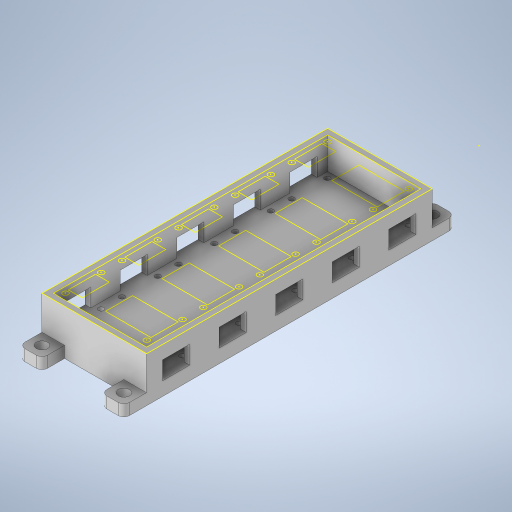
# Autodesk Inventor part: RelayCaseBottom
Saved by Autodesk Inventor 2024 (Build 280153000, 153)
## iProperties
Created: 2023-08-11
Part Number: RelayCaseBottom
Material: Generic
Document SubType Name: Modeling
Designer: 18179
Density: 1 g/cm^3
Appearance: Default
Autodesk Inventor part; units mm, degrees
ref_plane "YZ Plane" through (0, 0, 0) normal (1, 0, 0) x (0, 1, 0)
ref_plane "XZ Plane" through (0, 0, 0) normal (0, 1, 0) x (-1, 0, 0)
ref_plane "XY Plane" through (0, 0, 0) normal (0, 0, 1) x (1, 0, 0)
sketch "0" plane through (0, 0, 0) normal (0, 0, 1) x (1, 0, 0)
  line L0 (-39.8611, 34.3581) -> (-39.8611, 26.7381)
  line L1 (-39.8611, 26.7381) -> (-42.4011, 26.7381)
  line L2 (-42.4011, 26.7381) -> (-42.4011, 34.3581)
  line L3 (-42.4011, 34.3581) -> (-39.8611, 34.3581)
  line L4 (-37.9769, 46.974) -> (-63.3769, 46.974)
  line L5 (-63.3769, 46.974) -> (-63.3769, -3.826)
  line L6 (-63.3769, -3.826) -> (-37.9769, -3.826)
  line L7 (-37.9769, -3.826) -> (-37.9769, 46.974)
  line L8 (-58.2715, 6.588) -> (-58.2715, 24.368)
  line L9 (-58.2715, 24.368) -> (-43.0823, 24.368)
  line L10 (-43.0823, 24.368) -> (-43.0823, 6.588)
  line L11 (-43.0823, 6.588) -> (-43.0569, 6.588)
  line L12 (-43.0569, 6.588) -> (-43.0569, -1.159)
  line L13 (-43.0569, -1.159) -> (-58.2969, -1.159)
  line L14 (-58.2969, -1.159) -> (-58.2969, 6.588)
  line L15 (-58.2969, 6.588) -> (-58.2715, 6.588)
  line L16 (-58.2969, 37.449) -> (-58.2969, 45.196)
  line L17 (-58.2969, 45.196) -> (-43.0569, 45.196)
  line L18 (-43.0569, 45.196) -> (-43.0569, 37.449)
  line L19 (-43.0569, 37.449) -> (-58.2969, 37.449)
  circle A0 centre (-60.7099, -1.2407) radius 1.524
  circle A1 centre (-40.6439, -1.2407) radius 1.524
  circle A2 centre (-60.7099, 44.3888) radius 1.524
  circle A3 centre (-40.6439, 44.3888) radius 1.524
  line L20 (-71.6111, 34.3581) -> (-71.6111, 26.7381)
  line L21 (-71.6111, 26.7381) -> (-74.1511, 26.7381)
  line L22 (-74.1511, 26.7381) -> (-74.1511, 34.3581)
  line L23 (-74.1511, 34.3581) -> (-71.6111, 34.3581)
  line L24 (-69.7269, 46.974) -> (-95.1269, 46.974)
  line L25 (-95.1269, 46.974) -> (-95.1269, -3.826)
  line L26 (-95.1269, -3.826) -> (-69.7269, -3.826)
  line L27 (-69.7269, -3.826) -> (-69.7269, 46.974)
  line L28 (-90.0215, 6.588) -> (-90.0215, 24.368)
  line L29 (-90.0215, 24.368) -> (-74.8323, 24.368)
  line L30 (-74.8323, 24.368) -> (-74.8323, 6.588)
  line L31 (-74.8323, 6.588) -> (-74.8069, 6.588)
  line L32 (-74.8069, 6.588) -> (-74.8069, -1.159)
  line L33 (-74.8069, -1.159) -> (-90.0469, -1.159)
  line L34 (-90.0469, -1.159) -> (-90.0469, 6.588)
  line L35 (-90.0469, 6.588) -> (-90.0215, 6.588)
  line L36 (-90.0469, 37.449) -> (-90.0469, 45.196)
  line L37 (-90.0469, 45.196) -> (-74.8069, 45.196)
  line L38 (-74.8069, 45.196) -> (-74.8069, 37.449)
  line L39 (-74.8069, 37.449) -> (-90.0469, 37.449)
  circle A4 centre (-92.4599, -1.2407) radius 1.524
  circle A5 centre (-72.3939, -1.2407) radius 1.524
  circle A6 centre (-92.4599, 44.3888) radius 1.524
  circle A7 centre (-72.3939, 44.3888) radius 1.524
  line L40 (-103.3611, 34.3581) -> (-103.3611, 26.7381)
  line L41 (-103.3611, 26.7381) -> (-105.9011, 26.7381)
  line L42 (-105.9011, 26.7381) -> (-105.9011, 34.3581)
  line L43 (-105.9011, 34.3581) -> (-103.3611, 34.3581)
  line L44 (-101.4769, 46.974) -> (-126.8769, 46.974)
  line L45 (-126.8769, 46.974) -> (-126.8769, -3.826)
  line L46 (-126.8769, -3.826) -> (-101.4769, -3.826)
  line L47 (-101.4769, -3.826) -> (-101.4769, 46.974)
  line L48 (-121.7715, 6.588) -> (-121.7715, 24.368)
  line L49 (-121.7715, 24.368) -> (-106.5823, 24.368)
  line L50 (-106.5823, 24.368) -> (-106.5823, 6.588)
  line L51 (-106.5823, 6.588) -> (-106.5569, 6.588)
  line L52 (-106.5569, 6.588) -> (-106.5569, -1.159)
  line L53 (-106.5569, -1.159) -> (-121.7969, -1.159)
  line L54 (-121.7969, -1.159) -> (-121.7969, 6.588)
  line L55 (-121.7969, 6.588) -> (-121.7715, 6.588)
  line L56 (-121.7969, 37.449) -> (-121.7969, 45.196)
  line L57 (-121.7969, 45.196) -> (-106.5569, 45.196)
  line L58 (-106.5569, 45.196) -> (-106.5569, 37.449)
  line L59 (-106.5569, 37.449) -> (-121.7969, 37.449)
  circle A8 centre (-124.2099, -1.2407) radius 1.524
  circle A9 centre (-104.1439, -1.2407) radius 1.524
  circle A10 centre (-124.2099, 44.3888) radius 1.524
  circle A11 centre (-104.1439, 44.3888) radius 1.524
  line L60 (-135.1111, 34.3581) -> (-135.1111, 26.7381)
  line L61 (-135.1111, 26.7381) -> (-137.6511, 26.7381)
  line L62 (-137.6511, 26.7381) -> (-137.6511, 34.3581)
  line L63 (-137.6511, 34.3581) -> (-135.1111, 34.3581)
  line L64 (-133.2269, 46.974) -> (-158.6269, 46.974)
  line L65 (-158.6269, 46.974) -> (-158.6269, -3.826)
  line L66 (-158.6269, -3.826) -> (-133.2269, -3.826)
  line L67 (-133.2269, -3.826) -> (-133.2269, 46.974)
  line L68 (-153.5215, 6.588) -> (-153.5215, 24.368)
  line L69 (-153.5215, 24.368) -> (-138.3323, 24.368)
  line L70 (-138.3323, 24.368) -> (-138.3323, 6.588)
  line L71 (-138.3323, 6.588) -> (-138.3069, 6.588)
  line L72 (-138.3069, 6.588) -> (-138.3069, -1.159)
  line L73 (-138.3069, -1.159) -> (-153.5469, -1.159)
  line L74 (-153.5469, -1.159) -> (-153.5469, 6.588)
  line L75 (-153.5469, 6.588) -> (-153.5215, 6.588)
  line L76 (-153.5469, 37.449) -> (-153.5469, 45.196)
  line L77 (-153.5469, 45.196) -> (-138.3069, 45.196)
  line L78 (-138.3069, 45.196) -> (-138.3069, 37.449)
  line L79 (-138.3069, 37.449) -> (-153.5469, 37.449)
  circle A12 centre (-155.9599, -1.2407) radius 1.524
  circle A13 centre (-135.8939, -1.2407) radius 1.524
  circle A14 centre (-155.9599, 44.3888) radius 1.524
  circle A15 centre (-135.8939, 44.3888) radius 1.524
  line L80 (-166.8611, 34.3581) -> (-166.8611, 26.7381)
  line L81 (-166.8611, 26.7381) -> (-169.4011, 26.7381)
  line L82 (-169.4011, 26.7381) -> (-169.4011, 34.3581)
  line L83 (-169.4011, 34.3581) -> (-166.8611, 34.3581)
  line L84 (-164.9769, 46.974) -> (-190.3769, 46.974)
  line L85 (-190.3769, 46.974) -> (-190.3769, -3.826)
  line L86 (-190.3769, -3.826) -> (-164.9769, -3.826)
  line L87 (-164.9769, -3.826) -> (-164.9769, 46.974)
  line L88 (-185.2715, 6.588) -> (-185.2715, 24.368)
  line L89 (-185.2715, 24.368) -> (-170.0823, 24.368)
  line L90 (-170.0823, 24.368) -> (-170.0823, 6.588)
  line L91 (-170.0823, 6.588) -> (-170.0569, 6.588)
  line L92 (-170.0569, 6.588) -> (-170.0569, -1.159)
  line L93 (-170.0569, -1.159) -> (-185.2969, -1.159)
  line L94 (-185.2969, -1.159) -> (-185.2969, 6.588)
  line L95 (-185.2969, 6.588) -> (-185.2715, 6.588)
  line L96 (-185.2969, 37.449) -> (-185.2969, 45.196)
  line L97 (-185.2969, 45.196) -> (-170.0569, 45.196)
  line L98 (-170.0569, 45.196) -> (-170.0569, 37.449)
  line L99 (-170.0569, 37.449) -> (-185.2969, 37.449)
  circle A16 centre (-187.7099, -1.2407) radius 1.524
  circle A17 centre (-167.6439, -1.2407) radius 1.524
  circle A18 centre (-187.7099, 44.3888) radius 1.524
  circle A19 centre (-167.6439, 44.3888) radius 1.524
  line L100 (-37.9769, -3.826) -> (-190.3769, -3.826)
  line L101 (-190.3769, -3.826) -> (-190.3769, 46.974)
  line L102 (-190.3769, 46.974) -> (-37.9769, 46.974)
  line L103 (-37.9769, 46.974) -> (-37.9769, -3.826)
  line L104 (-190.3769, 47.736) -> (-37.2149, 47.736)
  line L105 (-37.2149, 47.736) -> (-37.2149, -3.826)
  line L106 (-37.9769, -4.588) -> (-191.1389, -4.588)
  line L107 (-191.1389, -4.588) -> (-191.1389, 46.974)
  line L108 (-191.1389, -4.588) -> (-37.2149, -4.588)
  line L109 (-37.2149, -4.588) -> (-37.2149, 47.736)
  line L110 (-37.2149, 47.736) -> (-191.1389, 47.736)
  line L111 (-191.1389, 47.736) -> (-191.1389, -4.588)
  point P0 (-37.2149, -3.826)
  dimension "d0" = 25.4
  dimension "d1" = 50.8
  dimension "d2" = 3.048
  dimension "d3" = 1.8843
  dimension "d4" = 4.4243
  dimension "d5" = 5.08
  dimension "d6" = 5.08
  dimension "d7" = 5.1054
  dimension "d8" = 20.2946
  dimension "d9" = 20.32
  dimension "d10" = 20.32
  dimension "d11" = 7.62
  dimension "d12" = 12.6159
  dimension "d13" = 10.8379
  dimension "d14" = 3.0909
  dimension "d15" = 9.9901
  dimension "d16" = 35.5171
  dimension "d17" = 27.7701
  dimension "d18" = 20.1501
  dimension "d19" = 12.6159
  dimension "d20" = 0
  dimension "d21" = 38.1841
  dimension "d22" = 0
  dimension "d23" = 0
  dimension "d24" = 1.8843
  dimension "d25" = 7.62
  dimension "d26" = 1.8843
  dimension "d27" = 2.667
  dimension "d28" = 10.0307
  dimension "d29" = 2.667
  dimension "d30" = 35.5988
  dimension "d31" = 0
  dimension "d32" = 4.4243
  dimension "d33" = 7.62
  dimension "d34" = 4.4243
  dimension "d35" = 10.8379
  dimension "d36" = 5.08
  dimension "d37" = 3.0909
  dimension "d38" = 5.08
  dimension "d39" = 5.08
  dimension "d40" = 27.7701
  dimension "d41" = 5.08
  dimension "d42" = 35.5171
  dimension "d43" = 9.9901
  dimension "d44" = 5.1054
  dimension "d45" = 5.1054
  dimension "d46" = 27.7701
  dimension "d47" = 9.9901
  dimension "d48" = 20.2946
  dimension "d49" = 27.7701
  dimension "d50" = 20.2946
  dimension "d51" = 10.8379
  dimension "d52" = 20.32
  dimension "d53" = 3.0909
  dimension "d54" = 20.32
  dimension "d55" = 20.32
  dimension "d56" = 27.7701
  dimension "d57" = 20.32
  dimension "d58" = 35.5171
  dimension "d59" = 22.733
  dimension "d60" = 10.0307
  dimension "d61" = 22.733
  dimension "d62" = 35.5988
  dimension "d63" = 25.4
  constraints: 224 end point, 44 parallel, 38 perpendicular, 20 centre point, 15 equal radius, 14 collinear, 2 horizontal, 2 other
  measures "d0" distance between parallel lines of L7 L5
  measures "d1" distance between parallel lines of L6 L4
  measures "d2" diameter of A3
  measures "d3" distance between parallel lines of L0 L7
  measures "d4" distance between parallel lines of L2 L7
  measures "d5" distance between parallel lines of L7 L18
  measures "d6" distance between parallel lines of L12 L7
  measures "d7" distance between parallel lines of L7 L10
  measures "d8" distance between parallel lines of L7 L8
  measures "d9" distance between parallel lines of L7 L16
  measures "d10" distance between parallel lines of L14 L7
  measures "d11" distance between parallel lines of L1 L3
  measures "d12" distance between parallel lines of L3 L4
  measures "d13" distance between parallel lines of L3 L17
  measures "d14" distance between parallel lines of L3 L19
  measures "d15" distance between parallel lines of L3 L9
  measures "d16" distance between parallel lines of L13 L3
  measures "d17" distance between parallel lines of L3 L15
  measures "d18" distance between parallel lines of L11 L1
  measures "d19" distance from line of L7.end L3
  measures "d20" distance from line of L4.start L7
  measures "d21" distance from line of L7.start L3
  measures "d22" distance from line of L6.end L7
  measures "d23" distance from line of L0.start L3
  measures "d24" distance from line of L3.end L7
  measures "d25" distance from line of L0.end L3
  measures "d26" distance from line of L1.start L7
  measures "d27" distance from line of A3.centre L7
  measures "d28" distance from line of A3.centre L3
  measures "d29" distance from line of A1.centre L7
  measures "d30" distance from line of A1.centre L3
  measures "d31" distance from line of L2.end L3
  measures "d32" distance from line of L3.start L7
  measures "d33" distance from line of L2.start L3
  measures "d34" distance from line of L1.end L7
  measures "d35" distance from line of L18.start L3
  measures "d36" distance from line of L17.end L7
  measures "d37" distance from line of L18.end L3
  measures "d38" distance from line of L19.start L7
  measures "d39" distance from line of L11.end L7
  measures "d40" distance from line of L12.start L3
  measures "d41" distance from line of L13.start L7
  measures "d42" distance from line of L12.end L3
  measures "d43" distance from line of L10.start L3
  measures "d44" distance from line of L9.end L7
  measures "d45" distance from line of L11.start L7
  measures "d46" distance from line of L10.end L3
  measures "d47" distance from line of L8.end L3
  measures "d48" distance from line of L9.start L7
  measures "d49" distance from line of L8.start L3
  measures "d50" distance from line of L15.end L7
  measures "d51" distance from line of L16.end L3
  measures "d52" distance from line of L17.start L7
  measures "d53" distance from line of L16.start L3
  measures "d54" distance from line of L19.end L7
  measures "d55" distance from line of L15.start L7
  measures "d56" distance from line of L14.end L3
  measures "d57" distance from line of L13.end L7
  measures "d58" distance from line of L14.start L3
  measures "d59" distance from line of A2.centre L7
  measures "d60" distance from line of A2.centre L3
  measures "d61" distance from line of A0.centre L7
  measures "d62" distance from line of A0.centre L3
  measures "d63" distance from line of L4.end L7
extrude "Extrusion1" add sketch "0" along normal blind 3.175 contours L0 L1 L2 L3 | L7 L6 L5 L4 | L5 L100 L27 L102 | L27 L26 L25 L24 | L25 L100 L47 L102 | L47 L46 L45 L44 | L45 L100 L67 L102 | L67 L66 L65 L64 | L65 L100 L87 L102 | L87 L86 L85 L84 | L20 L21 L22 L23 | L40 L41 L42 L43 | L60 L61 L62 L63 | L80 L81 L82 L83 | L104 L105 L109 L108 L106 L107 L111 L110
sketch "Sketch3" plane through (0, 0, 3.175) normal (0, 0, 1) x (1, 0, 0)
  line L0 (-191.1389, 47.736) -> (-191.1389, -4.588) projected
  line L1 (-191.1389, -4.588) -> (-37.2149, -4.588) projected
  line L2 (-37.2149, -4.588) -> (-37.2149, 47.736) projected
  line L3 (-37.2149, 47.736) -> (-191.1389, 47.736) projected
  line L4 (-58.2969, 37.449) -> (-58.2969, 45.196) projected
  line L5 (-58.2969, 45.196) -> (-43.0569, 45.196) projected
  line L6 (-43.0569, 45.196) -> (-43.0569, 37.449) projected
  line L7 (-43.0569, 37.449) -> (-58.2969, 37.449) projected
  circle A0 centre (-40.6439, 44.3888) radius 1.524 projected
  circle A1 centre (-60.7099, 44.3888) radius 1.524 projected
  circle A2 centre (-40.6439, -1.2407) radius 1.524 projected
  circle A3 centre (-60.7099, -1.2407) radius 1.524 projected
  line L8 (-106.5569, 37.449) -> (-121.7969, 37.449) projected
  line L9 (-121.7969, 37.449) -> (-121.7969, 45.196) projected
  line L10 (-121.7969, 45.196) -> (-106.5569, 45.196) projected
  line L11 (-106.5569, 45.196) -> (-106.5569, 37.449) projected
  circle A4 centre (-124.2099, 44.3888) radius 1.524 projected
  circle A5 centre (-104.1439, 44.3888) radius 1.524 projected
  circle A6 centre (-124.2099, -1.2407) radius 1.524 projected
  circle A7 centre (-104.1439, -1.2407) radius 1.524 projected
  circle A8 centre (-167.6439, -1.2407) radius 1.524 projected
  circle A9 centre (-187.7099, -1.2407) radius 1.524 projected
  circle A10 centre (-167.6439, 44.3888) radius 1.524 projected
  circle A11 centre (-187.7099, 44.3888) radius 1.524 projected
  line L12 (-170.0569, 37.449) -> (-185.2969, 37.449) projected
  line L13 (-185.2969, 37.449) -> (-185.2969, 45.196) projected
  line L14 (-185.2969, 45.196) -> (-170.0569, 45.196) projected
  line L15 (-170.0569, 45.196) -> (-170.0569, 37.449) projected
  line L16 (-185.2969, -1.159) -> (-185.2969, 6.588) projected
  line L17 (-185.2969, 6.588) -> (-185.2715, 6.588) projected
  line L18 (-185.2715, 6.588) -> (-185.2715, 24.368) projected
  line L19 (-185.2715, 24.368) -> (-170.0823, 24.368) projected
  line L20 (-170.0823, 24.368) -> (-170.0823, 6.588) projected
  line L21 (-170.0823, 6.588) -> (-170.0569, 6.588) projected
  line L22 (-170.0569, 6.588) -> (-170.0569, -1.159) projected
  line L23 (-170.0569, -1.159) -> (-185.2969, -1.159) projected
  circle A12 centre (-135.8939, -1.2407) radius 1.524 projected
  circle A13 centre (-155.9599, -1.2407) radius 1.524 projected
  circle A14 centre (-135.8939, 44.3888) radius 1.524 projected
  circle A15 centre (-155.9599, 44.3888) radius 1.524 projected
  line L24 (-138.3069, 37.449) -> (-153.5469, 37.449) projected
  line L25 (-153.5469, 37.449) -> (-153.5469, 45.196) projected
  line L26 (-153.5469, 45.196) -> (-138.3069, 45.196) projected
  line L27 (-138.3069, 45.196) -> (-138.3069, 37.449) projected
  circle A16 centre (-72.3939, -1.2407) radius 1.524 projected
  circle A17 centre (-92.4599, -1.2407) radius 1.524 projected
  circle A18 centre (-72.3939, 44.3888) radius 1.524 projected
  circle A19 centre (-92.4599, 44.3888) radius 1.524 projected
  line L28 (-74.8069, 37.449) -> (-90.0469, 37.449) projected
  line L29 (-90.0469, 37.449) -> (-90.0469, 45.196) projected
  line L30 (-90.0469, 45.196) -> (-74.8069, 45.196) projected
  line L31 (-74.8069, 45.196) -> (-74.8069, 37.449) projected
  line L32 (-194.3139, 50.911) -> (-194.3139, -7.763)
  line L33 (-194.3139, -7.763) -> (-34.0399, -7.763)
  line L34 (-34.0399, -7.763) -> (-34.0399, 50.911)
  line L35 (-34.0399, 50.911) -> (-194.3139, 50.911)
  line L36 (-185.2969, 45.196) -> (-170.0569, 45.196)
  line L37 (-170.0569, 45.196) -> (-170.0569, 50.911)
  line L38 (-170.0569, 50.911) -> (-185.2969, 50.911)
  line L39 (-185.2969, 50.911) -> (-185.2969, 45.196)
  line L40 (-153.5469, 45.196) -> (-138.3069, 45.196)
  line L41 (-138.3069, 45.196) -> (-138.3069, 50.911)
  line L42 (-138.3069, 50.911) -> (-153.5469, 50.911)
  line L43 (-153.5469, 50.911) -> (-153.5469, 45.196)
  line L44 (-121.7969, 45.196) -> (-106.5569, 45.196)
  line L45 (-106.5569, 45.196) -> (-106.5569, 50.911)
  line L46 (-106.5569, 50.911) -> (-121.7969, 50.911)
  line L47 (-121.7969, 50.911) -> (-121.7969, 45.196)
  line L48 (-90.0469, 45.196) -> (-74.8069, 45.196)
  line L49 (-74.8069, 45.196) -> (-74.8069, 50.911)
  line L50 (-74.8069, 50.911) -> (-90.0469, 50.911)
  line L51 (-90.0469, 50.911) -> (-90.0469, 45.196)
  line L52 (-58.2969, 45.196) -> (-43.0569, 45.196)
  line L53 (-43.0569, 45.196) -> (-43.0569, 50.911)
  line L54 (-43.0569, 50.911) -> (-58.2969, 50.911)
  line L55 (-58.2969, 50.911) -> (-58.2969, 45.196)
  line L56 (-185.2969, 50.911) -> (-170.0569, 50.911)
  line L57 (-170.0569, 50.911) -> (-170.0569, -7.763)
  line L58 (-170.0569, -7.763) -> (-185.2969, -7.763)
  line L59 (-185.2969, -7.763) -> (-185.2969, 50.911)
  line L60 (-153.5469, 50.911) -> (-138.3069, 50.911)
  line L61 (-138.3069, 50.911) -> (-138.3069, -7.763)
  line L62 (-138.3069, -7.763) -> (-153.5469, -7.763)
  line L63 (-153.5469, -7.763) -> (-153.5469, 50.911)
  line L64 (-121.7969, 50.911) -> (-106.5569, 50.911)
  line L65 (-106.5569, 50.911) -> (-106.5569, -7.763)
  line L66 (-106.5569, -7.763) -> (-121.7969, -7.763)
  line L67 (-121.7969, -7.763) -> (-121.7969, 50.911)
  line L68 (-90.0469, 50.911) -> (-74.8069, 50.911)
  line L69 (-74.8069, 50.911) -> (-74.8069, -7.763)
  line L70 (-74.8069, -7.763) -> (-90.0469, -7.763)
  line L71 (-90.0469, -7.763) -> (-90.0469, 50.911)
  line L72 (-58.2969, 50.911) -> (-43.0569, 50.911)
  line L73 (-43.0569, 50.911) -> (-43.0569, -7.763)
  line L74 (-43.0569, -7.763) -> (-58.2969, -7.763)
  line L75 (-58.2969, -7.763) -> (-58.2969, 50.911)
  point P0 (0, 0)
  point P1 (-153.5469, -4.588)
  point P2 (-170.0569, -4.588)
  point P3 (-121.7969, -4.588)
  point P4 (-138.3069, -4.588)
  point P5 (-90.0469, -4.588)
  point P6 (-106.5569, -4.588)
  point P7 (-58.2969, -4.588)
  point P8 (-74.8069, -4.588)
  point P9 (-43.0569, -4.588)
  point P10 (-43.0569, 47.736)
  point P11 (-58.2969, 47.736)
  point P12 (-74.8069, 47.736)
  point P13 (-90.0469, 47.736)
  point P14 (-106.5569, 47.736)
  point P15 (-121.7969, 47.736)
  point P16 (-138.3069, 47.736)
  point P17 (-153.5469, 47.736)
  point P18 (-170.0569, 47.736)
  point P19 (-185.2969, 47.736)
  point P20 (-185.2969, -4.588)
  dimension "d343" = 3.175
  constraints: 88 end point, 20 parallel, 10 horizontal, 10 perpendicular, 10 point on line, 3 other
  measures "d343" distance between parallel lines of L3 L35
extrude "Extrusion2" add sketch "Sketch3" along normal blind 10.16 contours L0 L1 L59 L33 L32 L35 L39 L3 | L37 L35 L43 L3 | L1 L63 L33 L57 | L41 L35 L47 L3 | L1 L67 L33 L61 | L45 L35 L51 L3 | L1 L71 L33 L65 | L49 L35 L55 L3 | L1 L75 L33 L69 | L53 L35 L34 L33 L73 L1 L2 L3
sketch "Sketch4" plane through (0, 0, 13.335) normal (0, 0, 1) x (1, 0, 0)
  line L0 (-37.2149, -4.588) -> (-43.0569, -4.588) projected
  line L1 (-43.0569, -4.588) -> (-43.0569, -7.763) projected
  line L2 (-43.0569, -7.763) -> (-34.0399, -7.763) projected
  line L3 (-34.0399, -7.763) -> (-34.0399, 50.911) projected
  line L4 (-34.0399, 50.911) -> (-43.0569, 50.911) projected
  line L5 (-43.0569, 50.911) -> (-43.0569, 47.736) projected
  line L6 (-43.0569, 47.736) -> (-37.2149, 47.736) projected
  line L7 (-37.2149, 47.736) -> (-37.2149, -4.588) projected
  line L8 (-58.2969, 50.911) -> (-74.8069, 50.911) projected
  line L9 (-58.2969, 50.911) -> (-74.8069, 50.911) projected
  line L10 (-74.8069, 50.911) -> (-74.8069, 47.736) projected
  line L11 (-74.8069, 47.736) -> (-58.2969, 47.736) projected
  line L12 (-58.2969, 47.736) -> (-58.2969, 50.911) projected
  line L13 (-90.0469, 50.911) -> (-106.5569, 50.911) projected
  line L14 (-106.5569, 50.911) -> (-106.5569, 47.736) projected
  line L15 (-106.5569, 47.736) -> (-90.0469, 47.736) projected
  line L16 (-90.0469, 47.736) -> (-90.0469, 50.911) projected
  line L17 (-90.0469, -4.588) -> (-106.5569, -4.588) projected
  line L18 (-106.5569, -4.588) -> (-106.5569, -7.763) projected
  line L19 (-106.5569, -7.763) -> (-90.0469, -7.763) projected
  line L20 (-90.0469, -7.763) -> (-90.0469, -4.588) projected
  line L21 (-58.2969, -4.588) -> (-74.8069, -4.588) projected
  line L22 (-74.8069, -4.588) -> (-74.8069, -7.763) projected
  line L23 (-74.8069, -7.763) -> (-58.2969, -7.763) projected
  line L24 (-58.2969, -7.763) -> (-58.2969, -4.588) projected
  line L25 (-121.7969, -4.588) -> (-138.3069, -4.588) projected
  line L26 (-138.3069, -4.588) -> (-138.3069, -7.763) projected
  line L27 (-138.3069, -7.763) -> (-121.7969, -7.763) projected
  line L28 (-121.7969, -7.763) -> (-121.7969, -4.588) projected
  line L29 (-121.7969, 50.911) -> (-138.3069, 50.911) projected
  line L30 (-138.3069, 50.911) -> (-138.3069, 47.736) projected
  line L31 (-138.3069, 47.736) -> (-121.7969, 47.736) projected
  line L32 (-121.7969, 47.736) -> (-121.7969, 50.911) projected
  line L33 (-153.5469, 50.911) -> (-170.0569, 50.911) projected
  line L34 (-170.0569, 50.911) -> (-170.0569, 47.736) projected
  line L35 (-170.0569, 47.736) -> (-153.5469, 47.736) projected
  line L36 (-153.5469, 47.736) -> (-153.5469, 50.911) projected
  line L37 (-191.1389, 47.736) -> (-185.2969, 47.736) projected
  line L38 (-185.2969, 47.736) -> (-185.2969, 50.911) projected
  line L39 (-185.2969, 50.911) -> (-194.3139, 50.911) projected
  line L40 (-194.3139, 50.911) -> (-194.3139, -7.763) projected
  line L41 (-194.3139, -7.763) -> (-185.2969, -7.763) projected
  line L42 (-185.2969, -7.763) -> (-185.2969, -4.588) projected
  line L43 (-185.2969, -4.588) -> (-191.1389, -4.588) projected
  line L44 (-191.1389, -4.588) -> (-191.1389, 47.736) projected
  line L45 (-153.5469, -4.588) -> (-170.0569, -4.588) projected
  line L46 (-170.0569, -4.588) -> (-170.0569, -7.763) projected
  line L47 (-170.0569, -7.763) -> (-153.5469, -7.763) projected
  line L48 (-153.5469, -7.763) -> (-153.5469, -4.588) projected
  line L49 (-185.2969, 47.736) -> (-170.0569, 47.736)
  line L50 (-170.0569, 47.736) -> (-170.0569, 50.911)
  line L51 (-170.0569, 50.911) -> (-185.2969, 50.911)
  line L52 (-185.2969, 50.911) -> (-185.2969, 47.736)
  line L53 (-153.5469, 47.736) -> (-138.3069, 47.736)
  line L54 (-138.3069, 47.736) -> (-138.3069, 50.911)
  line L55 (-138.3069, 50.911) -> (-153.5469, 50.911)
  line L56 (-153.5469, 50.911) -> (-153.5469, 47.736)
  line L57 (-121.7969, 47.736) -> (-106.5569, 47.736)
  line L58 (-106.5569, 47.736) -> (-106.5569, 50.911)
  line L59 (-106.5569, 50.911) -> (-121.7969, 50.911)
  line L60 (-121.7969, 50.911) -> (-121.7969, 47.736)
  line L61 (-106.5569, -4.588) -> (-121.7969, -4.588)
  line L62 (-121.7969, -4.588) -> (-121.7969, -7.763)
  line L63 (-121.7969, -7.763) -> (-106.5569, -7.763)
  line L64 (-106.5569, -7.763) -> (-106.5569, -4.588)
  line L65 (-138.3069, -4.588) -> (-153.5469, -4.588)
  line L66 (-153.5469, -4.588) -> (-153.5469, -7.763)
  line L67 (-153.5469, -7.763) -> (-138.3069, -7.763)
  line L68 (-138.3069, -7.763) -> (-138.3069, -4.588)
  line L69 (-170.0569, -4.588) -> (-185.2969, -4.588)
  line L70 (-185.2969, -4.588) -> (-185.2969, -7.763)
  line L71 (-185.2969, -7.763) -> (-170.0569, -7.763)
  line L72 (-170.0569, -7.763) -> (-170.0569, -4.588)
  line L73 (-43.0569, 47.736) -> (-58.2969, 47.736) projected
  line L74 (-43.0569, 50.911) -> (-58.2969, 50.911)
  line L75 (-58.2969, 50.911) -> (-58.2969, 47.736)
  line L76 (-58.2969, 47.736) -> (-43.0569, 47.736)
  line L77 (-43.0569, 47.736) -> (-43.0569, 50.911)
  line L78 (-74.8069, 47.736) -> (-90.0469, 47.736) projected
  line L79 (-74.8069, 50.911) -> (-90.0469, 50.911)
  line L80 (-90.0469, 50.911) -> (-90.0469, 47.736)
  line L81 (-90.0469, 47.736) -> (-74.8069, 47.736)
  line L82 (-74.8069, 47.736) -> (-74.8069, 50.911)
  line L83 (-43.0569, -4.588) -> (-58.2969, -4.588)
  line L84 (-58.2969, -4.588) -> (-58.2969, -7.763)
  line L85 (-58.2969, -7.763) -> (-43.0569, -7.763)
  line L86 (-43.0569, -7.763) -> (-43.0569, -4.588)
  line L87 (-74.8069, -4.588) -> (-90.0469, -4.588)
  line L88 (-90.0469, -4.588) -> (-90.0469, -7.763)
  line L89 (-90.0469, -7.763) -> (-74.8069, -7.763)
  line L90 (-74.8069, -7.763) -> (-74.8069, -4.588)
  point P0 (0, 0)
  constraints: 80 end point, 20 parallel, 10 horizontal, 10 perpendicular
extrude "Extrusion3" add sketch "Sketch4" along normal blind 7.62 contours L7 L6 L5 L4 L3 L2 L1 L0 | L1 L85 L24 L83 | L24 L23 L22 L21 | L73 L12 L74 L5 | L22 L89 L20 L87 | L11 L10 L8 L12 | L20 L19 L18 L17 | L78 L16 L79 L10 | L18 L63 L28 L61 | L15 L14 L13 L16 | L28 L27 L26 L25 | L57 L32 L59 L14 | L26 L67 L48 L65 | L31 L30 L29 L32 | L48 L47 L46 L45 | L53 L36 L55 L30 | L46 L71 L42 L69 | L35 L34 L33 L36 | L42 L41 L40 L39 L38 L37 L44 L43 | L49 L38 L51 L34
sketch "Sketch6" plane through (0, 0, 20.955) normal (0, 0, 1) x (1, 0, 0)
  line L0 (-191.1389, 47.736) -> (-191.1389, -4.588) projected
  line L1 (-191.1389, -4.588) -> (-185.2969, -4.588) projected
  line L2 (-185.2969, -4.588) -> (-170.0569, -4.588) projected
  line L3 (-170.0569, -4.588) -> (-153.5469, -4.588) projected
  line L4 (-153.5469, -4.588) -> (-138.3069, -4.588) projected
  line L5 (-138.3069, -4.588) -> (-121.7969, -4.588) projected
  line L6 (-121.7969, -4.588) -> (-106.5569, -4.588) projected
  line L7 (-106.5569, -4.588) -> (-90.0469, -4.588) projected
  line L8 (-90.0469, -4.588) -> (-74.8069, -4.588) projected
  line L9 (-74.8069, -4.588) -> (-58.2969, -4.588) projected
  line L10 (-58.2969, -4.588) -> (-43.0569, -4.588) projected
  line L11 (-43.0569, -4.588) -> (-37.2149, -4.588) projected
  line L12 (-37.2149, -4.588) -> (-37.2149, 47.736) projected
  line L13 (-37.2149, 47.736) -> (-43.0569, 47.736) projected
  line L14 (-43.0569, 47.736) -> (-58.2969, 47.736) projected
  line L15 (-58.2969, 47.736) -> (-74.8069, 47.736) projected
  line L16 (-74.8069, 47.736) -> (-90.0469, 47.736) projected
  line L17 (-90.0469, 47.736) -> (-106.5569, 47.736) projected
  line L18 (-106.5569, 47.736) -> (-121.7969, 47.736) projected
  line L19 (-121.7969, 47.736) -> (-138.3069, 47.736) projected
  line L20 (-138.3069, 47.736) -> (-153.5469, 47.736) projected
  line L21 (-153.5469, 47.736) -> (-170.0569, 47.736) projected
  line L22 (-170.0569, 47.736) -> (-185.2969, 47.736) projected
  line L23 (-185.2969, 47.736) -> (-191.1389, 47.736) projected
  line L24 (-90.0469, -1.159) -> (-90.0469, 6.588) projected
  line L25 (-90.0469, 6.588) -> (-90.0215, 6.588) projected
  line L26 (-90.0215, 6.588) -> (-90.0215, 24.368) projected
  line L27 (-90.0215, 24.368) -> (-74.8323, 24.368) projected
  line L28 (-74.8323, 24.368) -> (-74.8323, 6.588) projected
  line L29 (-74.8323, 6.588) -> (-74.8069, 6.588) projected
  line L30 (-74.8069, 6.588) -> (-74.8069, -1.159) projected
  line L31 (-74.8069, -1.159) -> (-90.0469, -1.159) projected
  line L32 (-74.8069, 37.449) -> (-90.0469, 37.449) projected
  line L33 (-90.0469, 37.449) -> (-90.0469, 45.196) projected
  line L34 (-90.0469, 45.196) -> (-74.8069, 45.196) projected
  line L35 (-74.8069, 45.196) -> (-74.8069, 37.449) projected
  circle A0 centre (-92.4599, 44.3888) radius 1.524 projected
  circle A1 centre (-72.3939, 44.3888) radius 1.524 projected
  circle A2 centre (-92.4599, -1.2407) radius 1.524 projected
  circle A3 centre (-72.3939, -1.2407) radius 1.524 projected
  line L36 (-153.5469, -1.159) -> (-153.5469, 6.588) projected
  line L37 (-153.5469, 6.588) -> (-153.5215, 6.588) projected
  line L38 (-153.5215, 6.588) -> (-153.5215, 24.368) projected
  line L39 (-153.5215, 24.368) -> (-138.3323, 24.368) projected
  line L40 (-138.3323, 24.368) -> (-138.3323, 6.588) projected
  line L41 (-138.3323, 6.588) -> (-138.3069, 6.588) projected
  line L42 (-138.3069, 6.588) -> (-138.3069, -1.159) projected
  line L43 (-138.3069, -1.159) -> (-153.5469, -1.159) projected
  line L44 (-138.3069, 37.449) -> (-153.5469, 37.449) projected
  line L45 (-153.5469, 37.449) -> (-153.5469, 45.196) projected
  line L46 (-153.5469, 45.196) -> (-138.3069, 45.196) projected
  line L47 (-138.3069, 45.196) -> (-138.3069, 37.449) projected
  circle A4 centre (-155.9599, 44.3888) radius 1.524 projected
  circle A5 centre (-135.8939, 44.3888) radius 1.524 projected
  circle A6 centre (-155.9599, -1.2407) radius 1.524 projected
  circle A7 centre (-135.8939, -1.2407) radius 1.524 projected
  line L48 (-185.2969, -1.159) -> (-185.2969, 6.588) projected
  line L49 (-185.2969, 6.588) -> (-185.2715, 6.588) projected
  line L50 (-185.2715, 6.588) -> (-185.2715, 24.368) projected
  line L51 (-185.2715, 24.368) -> (-170.0823, 24.368) projected
  line L52 (-170.0823, 24.368) -> (-170.0823, 6.588) projected
  line L53 (-170.0823, 6.588) -> (-170.0569, 6.588) projected
  line L54 (-170.0569, 6.588) -> (-170.0569, -1.159) projected
  line L55 (-170.0569, -1.159) -> (-185.2969, -1.159) projected
  line L56 (-170.0569, 37.449) -> (-185.2969, 37.449) projected
  line L57 (-185.2969, 37.449) -> (-185.2969, 45.196) projected
  line L58 (-185.2969, 45.196) -> (-170.0569, 45.196) projected
  line L59 (-170.0569, 45.196) -> (-170.0569, 37.449) projected
  circle A8 centre (-187.7099, 44.3888) radius 1.524 projected
  circle A9 centre (-167.6439, 44.3888) radius 1.524 projected
  circle A10 centre (-187.7099, -1.2407) radius 1.524 projected
  circle A11 centre (-167.6439, -1.2407) radius 1.524 projected
  circle A12 centre (-104.1439, -1.2407) radius 1.524 projected
  circle A13 centre (-124.2099, -1.2407) radius 1.524 projected
  circle A14 centre (-104.1439, 44.3888) radius 1.524 projected
  circle A15 centre (-124.2099, 44.3888) radius 1.524 projected
  line L60 (-106.5569, 37.449) -> (-121.7969, 37.449) projected
  line L61 (-121.7969, 37.449) -> (-121.7969, 45.196) projected
  line L62 (-121.7969, 45.196) -> (-106.5569, 45.196) projected
  line L63 (-106.5569, 45.196) -> (-106.5569, 37.449) projected
  line L64 (-121.7969, -1.159) -> (-121.7969, 6.588) projected
  line L65 (-121.7969, 6.588) -> (-121.7715, 6.588) projected
  line L66 (-121.7715, 6.588) -> (-121.7715, 24.368) projected
  line L67 (-121.7715, 24.368) -> (-106.5823, 24.368) projected
  line L68 (-106.5823, 24.368) -> (-106.5823, 6.588) projected
  line L69 (-106.5823, 6.588) -> (-106.5569, 6.588) projected
  line L70 (-106.5569, 6.588) -> (-106.5569, -1.159) projected
  line L71 (-106.5569, -1.159) -> (-121.7969, -1.159) projected
  line L72 (-58.2715, 6.588) -> (-58.2715, 24.368) projected
  line L73 (-58.2715, 24.368) -> (-43.0823, 24.368) projected
  line L74 (-43.0823, 24.368) -> (-43.0823, 6.588) projected
  line L75 (-43.0823, 6.588) -> (-43.0569, 6.588) projected
  line L76 (-43.0569, 6.588) -> (-43.0569, -1.159) projected
  line L77 (-43.0569, -1.159) -> (-58.2969, -1.159) projected
  line L78 (-58.2969, -1.159) -> (-58.2969, 6.588) projected
  line L79 (-58.2969, 6.588) -> (-58.2715, 6.588) projected
  line L80 (-58.2969, 37.449) -> (-58.2969, 45.196) projected
  line L81 (-58.2969, 45.196) -> (-43.0569, 45.196) projected
  line L82 (-43.0569, 45.196) -> (-43.0569, 37.449) projected
  line L83 (-43.0569, 37.449) -> (-58.2969, 37.449) projected
  circle A16 centre (-40.6439, 44.3888) radius 1.524 projected
  circle A17 centre (-60.7099, 44.3888) radius 1.524 projected
  circle A18 centre (-40.6439, -1.2407) radius 1.524 projected
  circle A19 centre (-60.7099, -1.2407) radius 1.524 projected
  line L84 (-34.0399, 50.911) -> (-194.3139, 50.911) projected
  line L85 (-194.3139, 50.911) -> (-194.3139, -7.763) projected
  line L86 (-194.3139, -7.763) -> (-34.0399, -7.763) projected
  line L87 (-34.0399, -7.763) -> (-34.0399, 50.911) projected
  line L88 (-191.1389, 47.736) -> (-37.2149, 47.736) projected
  line L89 (-37.2149, 47.736) -> (-37.2149, -4.588) projected
  line L90 (-37.2149, -4.588) -> (-191.1389, -4.588) projected
  line L91 (-191.1389, -4.588) -> (-191.1389, 47.736) projected
  point P0 (0, 0)
sketch "Sketch7" plane through (0, 0, 3.175) normal (0, 0, -1) x (-1, 0, 0)
  line L0 (194.3139, 50.911) -> (194.3139, -7.763) projected
  line L1 (194.3139, -7.763) -> (34.0399, -7.763) projected
  line L2 (194.3139, 50.911) -> (34.0399, 50.911)
  line L3 (34.0399, 50.911) -> (34.0399, -7.763)
  line L4 (34.0399, -7.763) -> (194.3139, -7.763)
  line L5 (194.3139, -7.763) -> (194.3139, 50.911)
  line L6 (191.1389, 47.736) -> (191.1389, -4.588) projected
  line L7 (37.2149, 47.736) -> (191.1389, 47.736)
  line L8 (191.1389, 47.736) -> (191.1389, -4.588)
  line L9 (191.1389, -4.588) -> (37.2149, -4.588)
  line L10 (37.2149, -4.588) -> (37.2149, 47.736)
  point P0 (0, 0)
  constraints: 16 end point, 4 parallel, 2 horizontal, 2 perpendicular
extrude "Extrusion4" add sketch "Sketch7" along normal blind 7.62
sketch "Sketch8" plane through (0, 0, -4.445) normal (0, 0, -1) x (-1, 0, 0)
  line L0 (194.3139, -7.763) -> (34.0399, -7.763) projected
  line L1 (34.0399, -7.763) -> (21.3399, -7.763)
  line L2 (21.3399, -7.763) -> (21.3399, 4.937)
  line L3 (21.3399, 4.937) -> (34.0399, 4.937)
  line L4 (34.0399, 4.937) -> (34.0399, -7.763)
  line L5 (194.3139, 50.911) -> (34.0399, 50.911) projected
  line L6 (34.0399, 50.911) -> (21.3399, 50.911)
  line L7 (21.3399, 50.911) -> (21.3399, 38.211)
  line L8 (21.3399, 38.211) -> (34.0399, 38.211)
  line L9 (34.0399, 38.211) -> (34.0399, 50.911)
  line L10 (194.3139, 50.911) -> (194.3139, -7.763) projected
  line L11 (194.3139, 50.911) -> (207.0139, 50.911)
  line L12 (207.0139, 50.911) -> (207.0139, 38.211)
  line L13 (207.0139, 38.211) -> (194.3139, 38.211)
  line L14 (194.3139, 38.211) -> (194.3139, 50.911)
  line L15 (194.3139, -7.763) -> (207.0139, -7.763)
  line L16 (207.0139, -7.763) -> (207.0139, 4.937)
  line L17 (207.0139, 4.937) -> (194.3139, 4.937)
  line L18 (194.3139, 4.937) -> (194.3139, -7.763)
  circle A0 centre (200.6639, -1.413) radius 3.175
  circle A1 centre (200.6639, 44.561) radius 3.175
  circle A2 centre (27.6899, 44.561) radius 3.175
  circle A3 centre (27.6899, -1.413) radius 3.175
  point P0 (0, 0)
  dimension "d350" = 12.7
  dimension "d351" = 12.7
  dimension "d352" = 12.7
  dimension "d353" = 12.7
  dimension "d354" = 12.7
  dimension "d355" = 12.7
  dimension "d356" = 12.7
  dimension "d357" = 12.7
  dimension "d358" = 6.35
  dimension "d359" = 6.35
  dimension "d360" = 6.35
  dimension "d361" = 6.35
  constraints: 32 end point, 8 parallel, 4 centre point, 4 horizontal, 4 perpendicular
  measures "d350" distance of L2.end L3.end
  measures "d351" distance of L1.end L2.end
  measures "d352" distance of L8.end L7.end
  measures "d353" distance of L7.end L6.end
  measures "d354" distance of L12.end L13.end
  measures "d355" distance of L11.end L12.end
  measures "d356" distance of L17.end L16.end
  measures "d357" distance of L16.end L15.end
  measures "d358" diameter of A0
  measures "d359" diameter of A1
  measures "d360" diameter of A2
  measures "d361" diameter of A3
extrude "Extrusion5" add sketch "Sketch8" against normal blind 6.35
fillet "Fillet1" radius 3.175 8 edges at (-207.0139, 38.211, -1.27) (-207.0139, 50.911, -1.27) (-207.0139, -7.763, -1.27) (-207.0139, 4.937, -1.27) (-21.3399, 50.911, -1.27) (-21.3399, 38.211, -1.27) (-21.3399, 4.937, -1.27) (-21.3399, -7.763, -1.27)
sketch "Sketch9" plane through (0, 0, 3.175) normal (0, 0, 1) x (1, 0, 0)
  line L0 (-191.1389, 47.736) -> (-191.1389, -4.588) projected
  line L1 (-191.1389, -4.588) -> (-185.2969, -4.588) projected
  line L2 (-185.2969, -7.763) -> (-185.2969, -4.588) projected
  line L3 (-170.0569, -7.763) -> (-185.2969, -7.763) projected
  line L4 (-170.0569, -4.588) -> (-170.0569, -7.763) projected
  line L5 (-170.0569, -4.588) -> (-153.5469, -4.588) projected
  line L6 (-153.5469, -7.763) -> (-153.5469, -4.588) projected
  line L7 (-138.3069, -7.763) -> (-153.5469, -7.763) projected
  line L8 (-138.3069, -4.588) -> (-138.3069, -7.763) projected
  line L9 (-138.3069, -4.588) -> (-121.7969, -4.588) projected
  line L10 (-121.7969, -7.763) -> (-121.7969, -4.588) projected
  line L11 (-106.5569, -7.763) -> (-121.7969, -7.763) projected
  line L12 (-106.5569, -4.588) -> (-106.5569, -7.763) projected
  line L13 (-106.5569, -4.588) -> (-90.0469, -4.588) projected
  line L14 (-90.0469, -7.763) -> (-90.0469, -4.588) projected
  line L15 (-74.8069, -7.763) -> (-90.0469, -7.763) projected
  line L16 (-74.8069, -4.588) -> (-74.8069, -7.763) projected
  line L17 (-74.8069, -4.588) -> (-58.2969, -4.588) projected
  line L18 (-58.2969, -7.763) -> (-58.2969, -4.588) projected
  line L19 (-43.0569, -7.763) -> (-58.2969, -7.763) projected
  line L20 (-43.0569, -4.588) -> (-43.0569, -7.763) projected
  line L21 (-43.0569, -4.588) -> (-37.2149, -4.588) projected
  line L22 (-37.2149, -4.588) -> (-37.2149, 47.736) projected
  line L23 (-37.2149, 47.736) -> (-43.0569, 47.736) projected
  line L24 (-43.0569, 50.911) -> (-43.0569, 47.736) projected
  line L25 (-58.2969, 50.911) -> (-43.0569, 50.911) projected
  line L26 (-58.2969, 47.736) -> (-58.2969, 50.911) projected
  line L27 (-58.2969, 47.736) -> (-74.8069, 47.736) projected
  line L28 (-74.8069, 50.911) -> (-74.8069, 47.736) projected
  line L29 (-90.0469, 50.911) -> (-74.8069, 50.911) projected
  line L30 (-90.0469, 47.736) -> (-90.0469, 50.911) projected
  line L31 (-90.0469, 47.736) -> (-106.5569, 47.736) projected
  line L32 (-106.5569, 50.911) -> (-106.5569, 47.736) projected
  line L33 (-121.7969, 50.911) -> (-106.5569, 50.911) projected
  line L34 (-121.7969, 47.736) -> (-121.7969, 50.911) projected
  line L35 (-121.7969, 47.736) -> (-138.3069, 47.736) projected
  line L36 (-138.3069, 50.911) -> (-138.3069, 47.736) projected
  line L37 (-153.5469, 50.911) -> (-138.3069, 50.911) projected
  line L38 (-153.5469, 47.736) -> (-153.5469, 50.911) projected
  line L39 (-153.5469, 47.736) -> (-170.0569, 47.736) projected
  line L40 (-170.0569, 50.911) -> (-170.0569, 47.736) projected
  line L41 (-185.2969, 50.911) -> (-170.0569, 50.911) projected
  line L42 (-185.2969, 47.736) -> (-185.2969, 50.911) projected
  line L43 (-185.2969, 47.736) -> (-191.1389, 47.736) projected
  line L44 (-90.0469, -1.159) -> (-90.0469, 6.588) projected
  line L45 (-90.0469, 6.588) -> (-90.0215, 6.588) projected
  line L46 (-90.0215, 6.588) -> (-90.0215, 24.368) projected
  line L47 (-90.0215, 24.368) -> (-74.8323, 24.368) projected
  line L48 (-74.8323, 24.368) -> (-74.8323, 6.588) projected
  line L49 (-74.8323, 6.588) -> (-74.8069, 6.588) projected
  line L50 (-74.8069, 6.588) -> (-74.8069, -1.159) projected
  line L51 (-74.8069, -1.159) -> (-90.0469, -1.159) projected
  line L52 (-74.8069, 37.449) -> (-90.0469, 37.449) projected
  line L53 (-90.0469, 37.449) -> (-90.0469, 45.196) projected
  line L54 (-90.0469, 45.196) -> (-74.8069, 45.196) projected
  line L55 (-74.8069, 45.196) -> (-74.8069, 37.449) projected
  circle A0 centre (-92.4599, 44.3888) radius 1.524 projected
  circle A1 centre (-72.3939, 44.3888) radius 1.524 projected
  circle A2 centre (-92.4599, -1.2407) radius 1.524 projected
  circle A3 centre (-72.3939, -1.2407) radius 1.524 projected
  line L56 (-153.5469, -1.159) -> (-153.5469, 6.588) projected
  line L57 (-153.5469, 6.588) -> (-153.5215, 6.588) projected
  line L58 (-153.5215, 6.588) -> (-153.5215, 24.368) projected
  line L59 (-153.5215, 24.368) -> (-138.3323, 24.368) projected
  line L60 (-138.3323, 24.368) -> (-138.3323, 6.588) projected
  line L61 (-138.3323, 6.588) -> (-138.3069, 6.588) projected
  line L62 (-138.3069, 6.588) -> (-138.3069, -1.159) projected
  line L63 (-138.3069, -1.159) -> (-153.5469, -1.159) projected
  line L64 (-138.3069, 37.449) -> (-153.5469, 37.449) projected
  line L65 (-153.5469, 37.449) -> (-153.5469, 45.196) projected
  line L66 (-153.5469, 45.196) -> (-138.3069, 45.196) projected
  line L67 (-138.3069, 45.196) -> (-138.3069, 37.449) projected
  circle A4 centre (-155.9599, 44.3888) radius 1.524 projected
  circle A5 centre (-135.8939, 44.3888) radius 1.524 projected
  circle A6 centre (-155.9599, -1.2407) radius 1.524 projected
  circle A7 centre (-135.8939, -1.2407) radius 1.524 projected
  line L68 (-185.2969, -1.159) -> (-185.2969, 6.588) projected
  line L69 (-185.2969, 6.588) -> (-185.2715, 6.588) projected
  line L70 (-185.2715, 6.588) -> (-185.2715, 24.368) projected
  line L71 (-185.2715, 24.368) -> (-170.0823, 24.368) projected
  line L72 (-170.0823, 24.368) -> (-170.0823, 6.588) projected
  line L73 (-170.0823, 6.588) -> (-170.0569, 6.588) projected
  line L74 (-170.0569, 6.588) -> (-170.0569, -1.159) projected
  line L75 (-170.0569, -1.159) -> (-185.2969, -1.159) projected
  line L76 (-170.0569, 37.449) -> (-185.2969, 37.449) projected
  line L77 (-185.2969, 37.449) -> (-185.2969, 45.196) projected
  line L78 (-185.2969, 45.196) -> (-170.0569, 45.196) projected
  line L79 (-170.0569, 45.196) -> (-170.0569, 37.449) projected
  circle A8 centre (-187.7099, 44.3888) radius 1.524 projected
  circle A9 centre (-167.6439, 44.3888) radius 1.524 projected
  circle A10 centre (-187.7099, -1.2407) radius 1.524 projected
  circle A11 centre (-167.6439, -1.2407) radius 1.524 projected
  circle A12 centre (-104.1439, -1.2407) radius 1.524 projected
  circle A13 centre (-124.2099, -1.2407) radius 1.524 projected
  circle A14 centre (-104.1439, 44.3888) radius 1.524 projected
  circle A15 centre (-124.2099, 44.3888) radius 1.524 projected
  line L80 (-106.5569, 37.449) -> (-121.7969, 37.449) projected
  line L81 (-121.7969, 37.449) -> (-121.7969, 45.196) projected
  line L82 (-121.7969, 45.196) -> (-106.5569, 45.196) projected
  line L83 (-106.5569, 45.196) -> (-106.5569, 37.449) projected
  line L84 (-121.7969, -1.159) -> (-121.7969, 6.588) projected
  line L85 (-121.7969, 6.588) -> (-121.7715, 6.588) projected
  line L86 (-121.7715, 6.588) -> (-121.7715, 24.368) projected
  line L87 (-121.7715, 24.368) -> (-106.5823, 24.368) projected
  line L88 (-106.5823, 24.368) -> (-106.5823, 6.588) projected
  line L89 (-106.5823, 6.588) -> (-106.5569, 6.588) projected
  line L90 (-106.5569, 6.588) -> (-106.5569, -1.159) projected
  line L91 (-106.5569, -1.159) -> (-121.7969, -1.159) projected
  line L92 (-58.2715, 6.588) -> (-58.2715, 24.368) projected
  line L93 (-58.2715, 24.368) -> (-43.0823, 24.368) projected
  line L94 (-43.0823, 24.368) -> (-43.0823, 6.588) projected
  line L95 (-43.0823, 6.588) -> (-43.0569, 6.588) projected
  line L96 (-43.0569, 6.588) -> (-43.0569, -1.159) projected
  line L97 (-43.0569, -1.159) -> (-58.2969, -1.159) projected
  line L98 (-58.2969, -1.159) -> (-58.2969, 6.588) projected
  line L99 (-58.2969, 6.588) -> (-58.2715, 6.588) projected
  line L100 (-58.2969, 37.449) -> (-58.2969, 45.196) projected
  line L101 (-58.2969, 45.196) -> (-43.0569, 45.196) projected
  line L102 (-43.0569, 45.196) -> (-43.0569, 37.449) projected
  line L103 (-43.0569, 37.449) -> (-58.2969, 37.449) projected
  circle A16 centre (-40.6439, 44.3888) radius 1.524 projected
  circle A17 centre (-60.7099, 44.3888) radius 1.524 projected
  circle A18 centre (-40.6439, -1.2407) radius 1.524 projected
  circle A19 centre (-60.7099, -1.2407) radius 1.524 projected
  point P0 (0, 0)
extrude "Extrusion6" add sketch "Sketch9" against normal blind 3.175 contours L44 L45 L46 L47 L48 L49 L50 L51 | L52 L53 L54 L55 | L56 L57 L58 L59 L60 L61 L62 L63 | L64 L65 L66 L67 | L68 L69 L70 L71 L72 L73 L74 L75 | L76 L77 L78 L79 | L80 L81 L82 L83 | L84 L85 L86 L87 L88 L89 L90 L91 | L92 L93 L94 L95 L96 L97 L98 L99 | L100 L101 L102 L103
body "Solid1"
